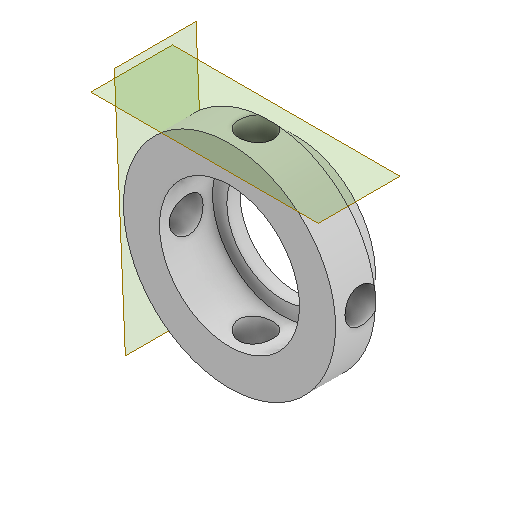
# Autodesk Inventor part: Tube_lens_holder
Saved by Autodesk Inventor 2023 (Build 270158000, 158)
## iProperties
Created: 2021-09-22
Part Number: Tube_lens_holder
Material: Generic
Document SubType Name: Modeling
Designer: CDT
Density: 1 g/cm^3
Appearance: Default
Author: CDT
Autodesk Inventor part; units mm, degrees
ref_plane "YZ Plane" through (0, 0, 0) normal (1, 0, 0) x (0, 1, 0)
ref_plane "XZ Plane" through (0, 0, 0) normal (0, 1, 0) x (-1, 0, 0)
ref_plane "XY Plane" through (0, 0, 0) normal (0, 0, 1) x (1, 0, 0)
sketch "Sketch1" plane through (0, 0, 0) normal (0, 0, 1) x (1, 0, 0)
  circle A0 centre (0, 0) radius 10
  circle A1 centre (0, 0) radius 6.6
  dimension "d0" = 20
  dimension "d1" = 13.2
  constraints: 2 centre point, 2 coincident
  measures "d0" diameter of A0
  measures "d1" diameter of A1
extrude "Extrusion1" add sketch "Sketch1" along normal blind 5
ref_plane "Work Plane2" through (0, 10, 0) normal (0, -1, 0) x (1, 0, 0)
ref_plane "Work Plane1" through (13.9005, -14, -0.9683) normal (0, -1, 0) x (1, 0, 0)
sketch "Sketch2" plane through (0, 10, 0) normal (0, -1, 0) x (1, 0, 0)
  circle A0 centre (0, 2.5) radius 1.6
  line L0 (10, 5) -> (-10, 5) projected
  line L1 (10, 0) -> (-10, 0) projected
  line L2 (-10, 0) -> (-10, 5) projected
  line L3 (0, 0) -> (-10, 0)
  line L4 (-10, 0) -> (-10, 3.2364)
  line L5 (-10, 3.2364) -> (0, 3.2364)
  line L6 (0, 3.2364) -> (0, 0)
  dimension "d4" = 3.2
  dimension "d7" = 2.5
  dimension "d8" = 2.5
  dimension "d16" = 10
  constraints: 8 end point, 2 parallel, 1 centre point, 1 horizontal, 1 perpendicular, 1 point on line
  measures "d4" diameter of A0
  measures "d7" distance from line of L0 A0.centre
  measures "d8" distance from line of L1 A0.centre
  measures "d16" distance from line of L2 A0.centre
extrude "Extrusion2" cut sketch "Sketch2" along normal through all contours A0 L6 L5 | L5 L6 A0
sketch "Sketch3" plane through (0, 0, 0) normal (0, 0, -1) x (-1, 0, 0)
  point P0 (0, 0)
sketch "Sketch4" plane through (0, 0, 0) normal (0, 0, -1) x (-1, 0, 0)
  circle A0 centre (0, 0) radius 10
  circle A1 centre (0, 0) radius 5.25
  dimension "d9" = 20
  dimension "d10" = 10.5
  constraints: 2 centre point, 2 coincident
  measures "d9" diameter of A0
  measures "d10" diameter of A1
extrude "Extrusion3" add sketch "Sketch4" along normal blind 1.25
chamfer "Chamfer1" distance 2.5 angle 45 1 edges at (10, 0, -1.25)
ref_plane "Work Plane4" through (-9.9898, -0.4509, 0) normal (-0.9989831, -0.0450859, 0) x (0.0450859, -0.9989831, 0)
ref_plane "Work Plane3" through (-24.6452, -6.2357, 39.5) normal (-0.9989831, -0.0450859, 0) x (0.0450859, -0.9989831, 0)
sketch "Sketch5" plane through (-9.9898, -0.4509, 0) normal (-0.9989831, -0.0450859, 0) x (0.0450859, -0.9989831, 0)
  circle A0 centre (0, 2.5) radius 1.6
  line L0 (10, 5) -> (-10, 5) projected
  point P0 (0, 0)
  dimension "d17" = 3.2
  dimension "d18" = 2.5
  constraints: 1 centre point
  measures "d17" diameter of A0
  measures "d18" distance from line of L0 A0.centre
extrude "Extrusion4" cut sketch "Sketch5" against normal blind 20
body "Solid1"
